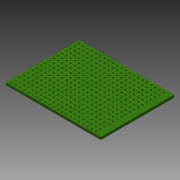
# Autodesk Inventor part: hextronik5744perfboard
Saved by Autodesk Inventor 2014 (Build 180170000, 170)
## iProperties
Created: 2014-05-21
Part Number: hextronik5744perfboard
Material: Generic
Document SubType Name: Modeling
Designer: brent
Density: 1 g/cm^3
Appearance: Default
Author: brent
Autodesk Inventor part; units mm, degrees
ref_plane "YZ Plane" through (0, 0, 0) normal (1, 0, 0) x (0, 1, 0)
ref_plane "XZ Plane" through (0, 0, 0) normal (0, 1, 0) x (-1, 0, 0)
ref_plane "XY Plane" through (0, 0, 0) normal (0, 0, 1) x (1, 0, 0)
sketch "Sketch1" plane through (0, 0, 0) normal (0, 1, 0) x (-1, 0, 0)
  line L0 (-33.3413, 19.976) -> (23.6587, 19.976)
  line L1 (23.6587, 19.976) -> (23.6587, -24.024)
  line L2 (23.6587, -24.024) -> (-33.3413, -24.024)
  line L3 (-33.3413, -24.024) -> (-33.3413, 19.976)
  point P0 (0, 0)
  dimension "d0" = 57
  dimension "d1" = 44
  constraints: 8 end point, 2 parallel, 1 horizontal, 1 perpendicular
  measures "d0" distance between parallel lines of L3 L1
  measures "d1" distance between parallel lines of L2 L0
extrude "Extrusion1" add sketch "Sketch1" along normal blind 1.5748
sketch "Sketch2" plane through (0, 1.5748, 0) normal (0, 1, 0) x (1, 0, 0)
  line L0 (33.3413, 24.024) -> (-23.6587, 24.024) projected
  line L1 (-23.6587, 24.024) -> (-23.6587, -19.976) projected
  circle A0 centre (-21.7537, 22.119) radius 0.5207
  point P0 (0, 0)
  dimension "d4" = 1.0414
  dimension "d5" = 1.905
  dimension "d6" = 1.905
  constraints: 1 centre point
  measures "d4" diameter of A0
  measures "d5" distance from line of L0 A0.centre
  measures "d6" distance from line of L1 A0.centre
extrude "Extrusion2" cut sketch "Sketch2" against normal through all
pattern_linear "Rectangular Pattern1" count 21 spacing 2.54 along (1, 0, 0) count 17 spacing 2.54 along (0, 0, 1) of "Extrusion2"
body "Solid1"
